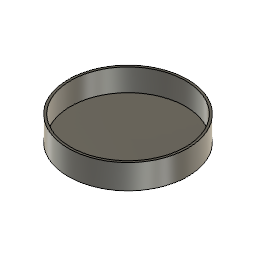
SchottflaschenHalterung (Autodesk Fusion 360 design; units mm, degrees)
part number: 2025-12-11-10-47-44-785
Autodesk Fusion 360 part; units mm, degrees
sketch "Skizze1" plane through (0, 0, 0) normal (0, 0, 1) x (1, 0, 0)
  circle A0 centre (0, 0) radius 53.5
  dimension "d1" = 107
  constraint coincident A0.centre origin
  measures "d1" diameter of A0
extrude "Extrusion1" add sketch "Skizze1" along normal blind 22
sketch "Skizze2" plane through (0, 0, 22) normal (0, 0, 1) x (-1, 0, 0)
  circle A0 centre (0, 0) radius 53.5
  circle A1 centre (0, 0) radius 51.5
  dimension "d4" = 103
  constraint coincident A0.centre A1.centre
  measures "d4" diameter of A1
extrude "Extrusion2" cut sketch "Skizze2" against normal blind 20 contours A1
